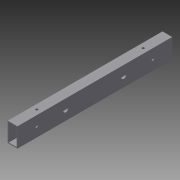
# Autodesk Inventor part: 000101
Saved by Autodesk Inventor 2015 (Build 190159000, 159)
## iProperties
Created: 2015-05-11
Part Number: 000101
Material: Generic
Document SubType Name: Modeling
Designer: Wesley
Density: 1 g/cm^3
Appearance: Default
Author: Wesley
Autodesk Inventor part; units mm, degrees
ref_plane "YZ Plane" through (0, 0, 0) normal (1, 0, 0) x (0, 1, 0)
ref_plane "XZ Plane" through (0, 0, 0) normal (0, 1, 0) x (-1, 0, 0)
ref_plane "XY Plane" through (0, 0, 0) normal (0, 0, 1) x (1, 0, 0)
sketch "Sketch1" plane through (0, 0, 0) normal (0, 0, 1) x (1, 0, 0)
  line L0 (0, 0) -> (12.7, 0)
  line L1 (12.7, 0) -> (12.7, 25.4)
  line L2 (12.7, 25.4) -> (0, 25.4)
  line L3 (0, 25.4) -> (0, 0)
  line L4 (1.27, 24.13) -> (11.43, 24.13)
  line L5 (11.43, 24.13) -> (11.43, 1.27)
  line L6 (11.43, 1.27) -> (1.27, 1.27)
  line L7 (1.27, 1.27) -> (1.27, 24.13)
  dimension "d0" = 25.4
  dimension "d1" = 12.7
  dimension "d2" = 1.27
  constraints: 16 end point, 4 parallel, 2 perpendicular, 1 horizontal, 3 other
  measures "d0" distance of L2.end L0.start
  measures "d1" distance of L0.start L0.end
  measures "d2" distance between parallel lines of L2 L4
extrude "Extrusion1" add sketch "Sketch1" along normal blind 203.2
sketch "Sketch2" plane through (12.7, 0, 0) normal (1, 0, 0) x (0, 0, -1)
  line L0 (-168.1044, 12.7) -> (-15.152, 12.7) construction
  line L1 (0, 0) -> (-203.2, 0) construction
  line L2 (-203.2, 0) -> (-203.2, 25.4) projected
  line L3 (0, 0) -> (0, 25.4) projected
  point P0 (-177.8, 12.7)
  point P1 (-25.4, 12.7)
  dimension "d5" = 12.7
  dimension "d6" = 25.4
  dimension "d7" = 25.4
  constraints: 2 end point, 2 point on line, 1 horizontal
  measures "d5" distance between parallel lines of L1 L0
  measures "d6" distance from line of L2 point (-177.8, 12.7)
  measures "d7" distance from line of L3 point (-25.4, 12.7)
hole "Hole1" at (12.7, 12.7, 177.8) at (12.7, 12.7, 25.4) direction (-1, 0, 0) diameter 3.2639 end through all
sketch "Sketch3" plane through (12.7, 0, 0) normal (1, 0, 0) x (0, 0, -1)
  circle A0 centre (-177.8, 12.7) radius 1.632 projected
  circle A1 centre (-25.4, 12.7) radius 1.632 projected
  line L0 (-214.4228, 12.7) -> (16.7128, 12.7) construction
  point P0 (0, 0)
  point P1 (-139.7, 12.7)
  point P2 (-63.5, 12.7)
  dimension "d18" = 38.1
  dimension "d19" = 38.1
  constraints: 2 coincident, 2 end point, 2 point on line, 1 horizontal
  measures "d18" distance of point (-177.8, 12.7) point (-139.7, 12.7)
  measures "d19" distance of point (-25.4, 12.7) point (-63.5, 12.7)
hole "Hole2" at (12.7, 12.7, 139.7) at (12.7, 12.7, 63.5) direction (-1, 0, 0) diameter 6.5278 end through all
sketch "Sketch4" plane through (0, 25.4, 0) normal (0, 1, 0) x (1, 0, 0)
  line L0 (6.35, 23.2485) -> (6.35, -226.9955) construction
  line L1 (12.7, 0) -> (12.7, -203.2) construction
  line L2 (12.7, 0) -> (0, 0) projected
  line L3 (0, 0) -> (0, -203.2) projected
  line L4 (12.7, -203.2) -> (0, -203.2) projected
  line L5 (12.7, 0) -> (12.7, -203.2) projected
  point P0 (0, 0)
  point P1 (6.35, -31.75)
  point P2 (6.35, -171.45)
  dimension "d27" = 6.35
  dimension "d28" = 31.75
  dimension "d29" = 31.75
  constraints: 2 end point, 2 point on line, 1 vertical
  measures "d27" distance between parallel lines of L1 L0
  measures "d28" distance from line of L2 point (6.35, -31.75)
  measures "d29" distance from line of L4 point (6.35, -171.45)
hole "Hole3" at (6.35, 25.4, 31.75) at (6.35, 25.4, 171.45) direction (0, -1, 0) diameter 3.2512 end through all
body "Solid1"
